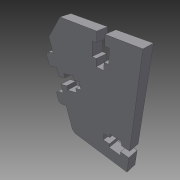
# Autodesk Inventor part: frame_brace_angled
Saved by Autodesk Inventor 2014 (Build 180170000, 170)
## iProperties
Created: 2014-03-31
Part Number: frame_brace_angled
Material: Generic
Document SubType Name: Modeling
Designer: buben
Density: 1 g/cm^3
Appearance: Default
Author: buben
Autodesk Inventor part; units mm, degrees
ref_plane "YZ Plane" through (0, 0, 0) normal (1, 0, 0) x (0, 1, 0)
ref_plane "XZ Plane" through (0, 0, 0) normal (0, 1, 0) x (-1, 0, 0)
ref_plane "XY Plane" through (0, 0, 0) normal (0, 0, 1) x (1, 0, 0)
sketch "Sketch1" plane through (0, 0, 0) normal (0, 1, 0) x (-1, 0, 0)
  line L0 (40.16, 0) -> (0, 0)
  line L1 (0, 0) -> (0, 67.5)
  line L2 (0, 67.5) -> (45, 67.5)
  line L3 (45, 67.5) -> (54.8252, 55)
  line L4 (54.8252, 55) -> (40.16, 0)
  dimension "d0" = 45
  dimension "d1" = 67.5
  dimension "d2" = 14.93
  dimension "d3" = 55
  dimension "d4" = 40.16
  constraints: 10 end point, 1 horizontal, 1 parallel, 1 perpendicular
  measures "d0" distance of L1.end L2.end
  measures "d1" distance of L0.end L1.end
  measures "d2" angle of L1 L4
  measures "d3" distance from line of L3.end L0
  measures "d4" distance of L0.start L0.end
extrude "Extrusion1" add sketch "Sketch1" along normal blind 6.5
chamfer "Chamfer1" distance 2 angle 45 1 edges at (-40.16, 3.25, 0)
sketch "Sketch2" plane through (0, 6.5, 0) normal (0, 1, 0) x (1, 0, 0)
  line L0 (-40.6753, -1.9325) -> (-54.8252, -55) projected
  line L1 (-45, -67.5) -> (0, -67.5) projected
  line L2 (0, -67.5) -> (0, 0) projected
  line L3 (0, 0) -> (-38.16, 0) projected
  line L4 (0, -10.75) -> (0, -15.25)
  line L5 (-16.3, -15.25) -> (-16.3, -10.75)
  line L6 (-12.3, -8.25) -> (-5, -8.25)
  line L7 (-5, -17.75) -> (-12.3, -17.75)
  line L8 (-16.3, -10.75) -> (-12.3, -10.75)
  line L9 (-5, -10.75) -> (0, -10.75)
  line L10 (0, -15.25) -> (-5, -15.25)
  line L11 (-12.3, -15.25) -> (-16.3, -15.25)
  line L12 (-12.3, -17.75) -> (-12.3, -15.25)
  line L13 (-12.3, -10.75) -> (-12.3, -8.25)
  line L14 (-5, -8.25) -> (-5, -10.75)
  line L15 (-5, -15.25) -> (-5, -17.75)
  line L16 (-49.2542, -34.1065) -> (-48.0948, -29.7584)
  line L17 (-32.3451, -33.958) -> (-33.5044, -38.306)
  line L18 (-38.0135, -39.6911) -> (-45.0671, -37.8103)
  line L19 (-42.6195, -28.631) -> (-35.5659, -30.5118)
  line L20 (-33.5044, -38.306) -> (-37.3694, -37.2755)
  line L21 (-44.423, -35.3947) -> (-49.2542, -34.1065)
  line L22 (-48.0948, -29.7584) -> (-43.2636, -31.0466)
  line L23 (-36.21, -32.9274) -> (-32.3451, -33.958)
  line L24 (-35.5659, -30.5118) -> (-36.21, -32.9274)
  line L25 (-37.3694, -37.2755) -> (-38.0135, -39.6911)
  line L26 (-45.0671, -37.8103) -> (-44.423, -35.3947)
  line L27 (-43.2636, -31.0466) -> (-42.6195, -28.631)
  line L28 (-17.75, -67.5) -> (-22.25, -67.5)
  line L29 (-22.25, -51.2) -> (-17.75, -51.2)
  line L30 (-15.25, -55.2) -> (-15.25, -62.5)
  line L31 (-24.75, -62.5) -> (-24.75, -55.2)
  line L32 (-17.75, -51.2) -> (-17.75, -55.2)
  line L33 (-17.75, -62.5) -> (-17.75, -67.5)
  line L34 (-22.25, -67.5) -> (-22.25, -62.5)
  line L35 (-22.25, -55.2) -> (-22.25, -51.2)
  line L36 (-24.75, -55.2) -> (-22.25, -55.2)
  line L37 (-17.75, -55.2) -> (-15.25, -55.2)
  line L38 (-15.25, -62.5) -> (-17.75, -62.5)
  line L39 (-22.25, -62.5) -> (-24.75, -62.5)
  point P0 (-32.9247, -36.132)
  point P1 (-20, -51.2)
  point P2 (-48.6745, -31.9325)
  point P3 (-16.3, -13)
  dimension "d10" = 4.5
  dimension "d11" = 4
  dimension "d12" = 5
  dimension "d13" = 7.3
  dimension "d14" = 2.5
  dimension "d15" = 4.5
  dimension "d16" = 4
  dimension "d17" = 5
  dimension "d18" = 7.3
  dimension "d19" = 2.5
  dimension "d20" = 4.5
  dimension "d21" = 4
  dimension "d22" = 5
  dimension "d23" = 7.3
  dimension "d24" = 2.5
  dimension "d25" = 30
  dimension "d26" = 20
  dimension "d27" = 13
  constraints: 72 end point, 32 parallel, 18 collinear, 12 perpendicular, 4 midpoint, 3 horizontal
  measures "d10" distance of L5.start L5.end
  measures "d11" distance of L5.end L8.end
  measures "d12" distance of L9.start L4.start
  measures "d13" distance of L6.start L6.end
  measures "d14" distance of L8.end L6.start
  measures "d15" distance of L17.start L20.start
  measures "d16" distance of L20.start L25.start
  measures "d17" distance of L26.end L16.start
  measures "d18" distance of L18.start L26.start
  measures "d19" distance of L25.start L18.start
  measures "d20" distance of L29.start L32.start
  measures "d21" distance of L32.start L37.start
  measures "d22" distance of L38.end L28.start
  measures "d23" distance of L30.start L38.start
  measures "d24" distance of L37.start L30.start
  measures "d25" vertical distance of L0.start point (-48.674, -31.932)
  measures "d26" distance from line of L2 point (-20, -51.2)
  measures "d27" distance from line of point (-16.3, -13) L3
extrude "Extrusion2" cut sketch "Sketch2" against normal through all
sketch "Sketch3" plane through (0, 6.5, 0) normal (0, 1, 0) x (1, 0, 0)
  line L0 (-32.3451, -33.958) -> (-33.5044, -38.306) projected
  line L1 (-49.2542, -34.1065) -> (-54.8252, -55) projected
  line L2 (-40.6753, -1.9325) -> (-48.0948, -29.7584) projected
  line L3 (-44.6811, -16.9557) -> (-46.7422, -24.6857)
  line L4 (-46.7422, -24.6857) -> (-51.0903, -23.5263)
  line L5 (-52.5075, -21.0785) -> (-51.4769, -17.2136)
  line L6 (-49.0292, -15.7964) -> (-44.6811, -16.9557)
  line L7 (-50.6068, -39.1793) -> (-52.6679, -46.9092)
  line L8 (-52.6679, -46.9092) -> (-57.016, -45.7498)
  line L9 (-58.4332, -43.3021) -> (-57.4026, -39.4371)
  line L10 (-54.9549, -38.0199) -> (-50.6068, -39.1793)
  arc A0 (-49.0292, -15.7964) -> (-51.4769, -17.2136) centre (-49.5444, -17.7289) ccw
  arc A1 (-52.5075, -21.0785) -> (-51.0903, -23.5263) centre (-50.575, -21.5938) ccw
  arc A2 (-54.9549, -38.0199) -> (-57.4026, -39.4371) centre (-55.4701, -39.9524) ccw
  arc A3 (-58.4332, -43.3021) -> (-57.016, -45.7498) centre (-56.5007, -43.8174) ccw
  point P0 (-32.9247, -36.132)
  dimension "d30" = 2
  dimension "d31" = 8
  dimension "d32" = 8
  dimension "d33" = 15
  dimension "d34" = 7.5
  dimension "d35" = 6.5
  constraints: 16 end point, 8 point on circle, 8 tangent, 4 centre point, 4 parallel, 4 point on line, 3 equal radius, 2 perpendicular, 1 collinear, 1 midpoint
  measures "d30" radius of A0
  measures "d31" distance between parallel lines of L4 L6
  measures "d32" distance between parallel lines of L8 L10
  measures "d33" distance between parallel lines of L10 L4
  measures "d34" distance from line of point (-32.925, -36.132) L4
  measures "d35" distance between parallel lines of L2 L5
extrude "Extrusion3" add sketch "Sketch3" against normal blind 6.5
equation "\"d32\" = d31"
equation "\"d34\" = 0.5 * d33"
body "Solid1"
